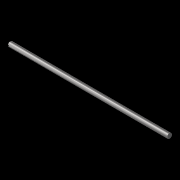
# Autodesk Inventor part: Axle
Saved by Autodesk Inventor 2018 (Build 220112000, 112)
## iProperties
Created: 2022-03-30
Part Number: Axle
Material: Steel, Carbon
Document SubType Name: Modeling
Designer: kumpu
Density: 7.85 g/cm^3
Appearance: Semi-Polished
Author: kumpu
Autodesk Inventor part; units mm, degrees
ref_plane "YZ Plane" through (0, 0, 0) normal (1, 0, 0) x (0, 1, 0)
ref_plane "XZ Plane" through (0, 0, 0) normal (0, 1, 0) x (-1, 0, 0)
ref_plane "XY Plane" through (0, 0, 0) normal (0, 0, 1) x (1, 0, 0)
sketch "Sketch1" plane through (0, 0, 0) normal (1, 0, 0) x (0, 1, 0)
  arc A0 (-1.5875, 6.1484) -> (1.5875, 6.1484) centre (0, 0) ccw
  line L0 (-1.5875, 6.1484) -> (-1.5875, 4.7498)
  line L1 (-1.5875, 4.7498) -> (1.5875, 4.7498)
  line L2 (1.5875, 4.7498) -> (1.5875, 6.1484)
  line L3 (-1.5875, 4.7498) -> (1.5875, 4.7498) construction
  line L4 (1.5875, 4.7498) -> (1.5875, 6.35) construction
  line L5 (1.5875, 6.35) -> (-1.5875, 6.35) construction
  line L6 (-1.5875, 6.35) -> (-1.5875, 4.7498) construction
  dimension "d0" = 1.6002
  dimension "d1" = 3.175
  dimension "d2" = 6.35
  constraints: 14 end point, 3 parallel, 3 perpendicular, 2 point on circle, 1 centre point, 1 coincident, 1 collinear, 1 horizontal, 1 tangent, 1 vertical
  measures "d0" distance of L3.end L4.end
  measures "d1" distance of L0.end L1.end
  measures "d2" radius of A0
extrude "Extrusion1" add sketch "Sketch1" along normal blind 406.4
body "Solid1"
